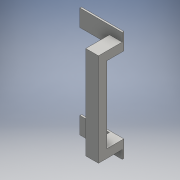
# Autodesk Inventor part: servobridge
Saved by Autodesk Inventor 2016 (Build 200138000, 138)
## iProperties
Created: 2016-04-09
Part Number: servobridge
Material: Generic
Document SubType Name: Modeling
Designer: kmonte
Density: 1 g/cm^3
Appearance: Default
Author: kmonte
Autodesk Inventor part; units mm, degrees
ref_plane "YZ Plane" through (0, 0, 0) normal (1, 0, 0) x (0, 1, 0)
ref_plane "XZ Plane" through (0, 0, 0) normal (0, 1, 0) x (-1, 0, 0)
ref_plane "XY Plane" through (0, 0, 0) normal (0, 0, 1) x (1, 0, 0)
sketch "Sketch1" plane through (0, 0, 0) normal (0, 1, 0) x (-1, 0, 0)
  line L0 (0, 0) -> (15, 0)
  line L1 (15, 0) -> (15, -110)
  line L2 (15, -110) -> (0, -110)
  line L3 (0, -110) -> (0, 0)
  dimension "d0" = 110
  dimension "d1" = 15
  constraints: 8 end point, 2 parallel, 1 horizontal, 1 perpendicular
  measures "d0" distance of L0.end L1.end
  measures "d1" distance of L1.end L2.end
extrude "Extrusion1" add sketch "Sketch1" along normal blind 10
sketch "Sketch2" plane through (0, 10, 0) normal (0, 1, 0) x (1, 0, 0)
  line L0 (-15, 0) -> (0, 0) projected
  line L1 (0, 0) -> (0, 110) projected
  line L2 (-15, 0) -> (0, 0)
  line L3 (0, 0) -> (0, 10)
  line L4 (0, 10) -> (-15, 10)
  line L5 (-15, 10) -> (-15, 0)
  line L6 (0, 110) -> (-15, 110) projected
  line L7 (-15, 110) -> (0, 110)
  line L8 (0, 110) -> (0, 100)
  line L9 (0, 100) -> (-15, 100)
  line L10 (-15, 100) -> (-15, 110)
  dimension "d4" = 10
  dimension "d5" = 10
  constraints: 16 end point, 4 parallel, 2 horizontal, 2 perpendicular, 2 point on line
  measures "d4" distance of L4.end L0.start
  measures "d5" distance of L9.end L6.end
extrude "Extrusion2" add sketch "Sketch2" along normal blind 18
sketch "Sketch3" plane through (0, 28, 0) normal (0, 1, 0) x (1, 0, 0)
  line L0 (0, 0) -> (0, 10) projected
  line L1 (0, 10) -> (-50, 10)
  line L2 (-50, 10) -> (-50, -10)
  line L3 (-50, -10) -> (0, -10)
  line L4 (0, -10) -> (0, 10)
  line L5 (-15, 100) -> (0, 100) projected
  line L6 (0, 100) -> (-50, 100)
  line L7 (-50, 100) -> (-50, 120)
  line L8 (-50, 120) -> (0, 120)
  line L9 (0, 120) -> (0, 100)
  dimension "d8" = 50
  dimension "d9" = 20
  dimension "d10" = 50
  dimension "d11" = 20
  constraints: 16 end point, 4 parallel, 2 horizontal, 2 perpendicular
  measures "d8" distance of L3.end L2.end
  measures "d9" distance of L1.end L2.end
  measures "d10" distance of L7.end L8.end
  measures "d11" distance of L6.end L7.end
extrude "Extrusion3" add sketch "Sketch3" along normal blind 2
body "Solid1"
